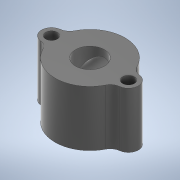
# Autodesk Inventor part: BearingHolderInlet
Saved by Autodesk Inventor 2020.2 (Build 242310000, 310)
## iProperties
Created: 2020-10-21
Part Number: BearingHolderInlet
Material: Generic
Document SubType Name: Modeling
Designer: JK
Density: 1 g/cm^3
Appearance: Smooth - Black
Author: JK
Autodesk Inventor part; units mm, degrees
ref_plane "YZ Plane" through (0, 0, 0) normal (1, 0, 0) x (0, 1, 0)
ref_plane "XZ Plane" through (0, 0, 0) normal (0, 1, 0) x (-1, 0, 0)
ref_plane "XY Plane" through (0, 0, 0) normal (0, 0, 1) x (1, 0, 0)
sketch "Sketch1" plane through (0, 0, 0) normal (0, 1, 0) x (-1, 0, 0)
  circle A0 centre (0, 0) radius 13.35
  circle A1 centre (0, 0) radius 16.35
  dimension "d0" = 26.7
  dimension "d1" = 3
  constraints: 2 centre point, 2 coincident
  measures "d0" diameter of A0
  measures "d1" radial gap between concentric circles of A1 A0
extrude "Extrusion1" add sketch "Sketch1" along normal blind 8
sketch "Sketch2" plane through (0, 8, 0) normal (0, 1, 0) x (1, 0, 0)
  circle A0 centre (0, 0) radius 16.35 projected
  circle A1 centre (0, 0) radius 13.35 projected
  circle A2 centre (0, 0) radius 6.75
  dimension "d4" = 13.5
  constraints: 1 centre point, 1 coincident
  measures "d4" diameter of A2
extrude "Extrusion2" add sketch "Sketch2" along normal blind 2 contours A0 | A1
sketch "Sketch5" plane through (0, 0, 0) normal (0, -1, 0) x (1, 0, 0)
  circle A0 centre (18, 0) radius 2.75
  circle A1 centre (-18, 0) radius 2.75
  circle A2 centre (18, 0) radius 4.65
  circle A3 centre (0, 0) radius 13.35 projected
  circle A4 centre (-18, 0) radius 4.65
  dimension "d19" = 18
  dimension "d20" = 18
  dimension "d21" = 5.5
  dimension "d22" = 5.5
  constraints: 4 centre point, 2 coincident, 2 tangent
  measures "d19" distance of point (0, 0) A0.centre
  measures "d20" distance of A1.centre point (0, 0)
  measures "d21" diameter of A0
  measures "d22" diameter of A1
extrude "Extrusion5" add sketch "Sketch5" against normal up to surface (10 mm away) contours A2 | A4
sketch "Sketch6" plane through (0, 0, 0) normal (0, -1, 0) x (1, 0, 0)
  arc A0 (16.2156, -2.0924) -> (16.2156, 2.0924) centre (18, 0) ccw projected
  circle A1 centre (18, 0) radius 2.75
  arc A2 (-16.2156, 2.0924) -> (-16.2156, -2.0924) centre (-18, 0) ccw projected
  circle A3 centre (-18, 0) radius 2.75
  point P0 (0, 0)
  point P1 (-16.2156, -2.0924)
  point P2 (16.2156, 2.0924)
  constraints: 2 centre point, 2 coincident
extrude "Extrusion6" cut sketch "Sketch6" against normal through all
sketch "Sketch7" plane through (0, 10, 0) normal (0, 1, 0) x (1, 0, 0)
  arc A0 (-15.825, 4.11) -> (-15.825, -4.11) centre (-18, 0) ccw projected
  arc A1 (-15.825, -4.11) -> (15.825, -4.11) centre (0, 0) ccw projected
  arc A2 (15.825, -4.11) -> (15.825, 4.11) centre (18, 0) ccw projected
  arc A3 (15.825, 4.11) -> (-15.825, 4.11) centre (0, 0) ccw projected
  circle A4 centre (0, 0) radius 6.75 projected
  circle A5 centre (-18, 0) radius 2.75 projected
  circle A6 centre (18, 0) radius 2.75 projected
extrude "Extrusion7" add sketch "Sketch7" along normal blind 16
sketch "Sketch8" plane through (0, 0, 0) normal (0, 0, 1) x (1, 0, 0)
  circle A0 centre (0, 16) radius 6.75
  line L0 (15.825, 0) -> (-15.825, 0) projected
  point P0 (0, 0)
  point P1 (0, 0)
  dimension "d29" = 13.5
  dimension "d30" = 16
  constraints: 1 centre point, 1 midpoint, 1 vertical alignment
  measures "d29" diameter of A0
  measures "d30" distance from line of A0.centre L0
extrude "Extrusion8" cut sketch "Sketch8" against normal through all
fillet "Fillet1" radius 5 7 edges at (-15.825, 18, -4.11) (-15.825, 5, -4.11) (-15.825, 18, 4.11) (-15.825, 5, 4.11) (15.825, 18, 4.11) (15.825, 5, 4.11) (15.825, 13, -4.11)
body "Solid1"
